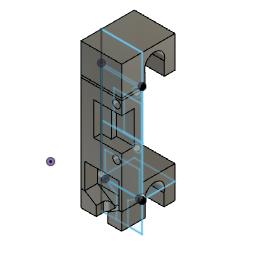
X Stop-block (Autodesk Fusion 360 design; units mm, degrees)
Autodesk Fusion 360 part; units mm, degrees
sketch "Sketch1" plane through (0, 0, 0) normal (1, 0, 0) x (0, 1, 0) in component "Component"
  line L0 (0, 0) -> (1, 0)
  line L1 (1, 0) -> (1, 40)
  line L2 (1, 40) -> (0, 40)
  line L3 (0, 40) -> (0, 0)
  dimension "d3" = 1
  dimension "d4" = 40
  constraint horizontal L0
  constraint vertical L1
  constraint horizontal L2
  constraint vertical L3
  constraint coincident L0.start L3.end
  measures "d3" distance of L0.start L0.end
  measures "d4" distance of L0.start L2.end
extrude "Extrude1" add sketch "Sketch1" against normal blind 20 makes body 1 in component "Component"
sketch "Sketch2" plane through (0, 1, 0) normal (0, 1, 0) x (-1, 0, 0) in component "Component"
  line L0 (0, 40) -> (0, 0)
  line L1 (0, 0) -> (20, 0)
  line L2 (20, 0) -> (20, 40)
  line L3 (20, 40) -> (0, 40)
  line L4 (6.0137, 29.6802) -> (6.0137, 12.583)
  line L5 (14.1333, 29.3642) -> (14.1333, 12.3406)
  arc A0 (14.1333, 29.3642) -> (6.0137, 29.6802) centre (10.1692, 31.9811) ccw
  line L6 (5.8481, 7.6926) -> (5.8481, 0)
  line L7 (13.9529, 7.3662) -> (13.9529, 0)
  arc A1 (6.0137, 12.583) -> (5.8481, 7.6926) centre (10, 10) ccw
  arc A2 (13.9529, 7.3662) -> (14.1333, 12.3406) centre (10, 10) ccw
  point P0 (10, 10)
  dimension "d7" = 9.5
  dimension "d8" = 9.5
  constraint coincident P0 A1.centre
  constraint vertical L4
  constraint parallel L2 L5
  constraint coincident L1 L6.end
  constraint perpendicular L1 L6
  constraint coincident L7.start A1
  constraint coincident L1 L7.end
  constraint perpendicular L1 L7
  constraint concentric A1 A2
  measures "d7" diameter of A0
  measures "d8" diameter of A1
extrude "Extrude2" cut sketch "Sketch2" against normal up to surface (1 mm away) contours L1 L4 L5 A0 L6 L7 A1 A2 bodies 1 in component "Component"
extrude "Extrude3" add 1 faces at (-18.2048, 0, 17.0423) along direction (0, -1, 0) blind 4 on bodies 1 bodies 1 in component "Component"
extrude "Extrude4" add 1 faces at (-20, -2.3333, 26.6667) along direction (-1, 0, 0) blind 13 on bodies 1 bodies 1 in component "Component"
sketch "Sketch3" plane through (0, 0, 40) normal (0, 0, 1) x (-1, 0, 0)
  line L0 (0, 4) -> (0, -1)
  line L1 (0, -1) -> (33, -1)
  line L2 (33, -1) -> (33, 4)
  line L3 (33, 4) -> (0, 4)
  line L4 (33, -1) -> (17, -1)
  line L5 (17, -1) -> (17, 4)
  line L6 (17, 4) -> (33, 4)
  line L7 (33, 4) -> (33, -1)
  dimension "d16" = 16
  constraint horizontal L4
  constraint vertical L5
  constraint horizontal L6
  constraint vertical L7
  constraint coincident L1.end L2.start
  measures "d16" distance of L1.end L4.end
extrude "Extrude5" add sketch "Sketch3" along normal blind 28 contours L1 L2 L3 L4 L5 L6 L7 bodies 1 in component "Component"
sketch "Sketch4" plane through (0, -4, 0) normal (0, -1, 0) x (1, 0, 0)
  line L0 (-13.9529, 0) -> (-13.9529, 7.3662)
  arc A0 (-14.1333, 12.3406) -> (-13.9529, 7.3662) centre (-10, 10) ccw
  line L1 (-14.1333, 12.3406) -> (-14.1333, 29.3642)
  arc A1 (-6.0137, 29.6802) -> (-14.1333, 29.3642) centre (-10.1692, 31.9811) ccw
  line L2 (-6.0137, 29.6802) -> (-6.0137, 12.583)
  arc A2 (-5.8481, 7.6926) -> (-6.0137, 12.583) centre (-10, 10) ccw
  line L3 (-5.8481, 7.6926) -> (-5.8481, 0)
  line L4 (-5.8481, 0) -> (0, 0)
  line L5 (0, 0) -> (0, 40)
  line L6 (0, 40) -> (-17, 40)
  line L7 (-17, 40) -> (-17, 68)
  line L8 (-17, 68) -> (-33, 68)
  line L9 (-33, 68) -> (-33, 0)
  line L10 (-33, 0) -> (-13.9529, 0)
  line L11 (-20, 0) -> (-20, 20)
  line L12 (-20, 20) -> (-33, 29.3642)
  line L13 (-33, 0) -> (-20, 0)
  line L14 (-33, 29.3642) -> (-33, 0)
  constraint coincident L10 L11.start
  constraint perpendicular L10 L11
  constraint coincident L9 L12.end
  constraint coincident L9.end L10.start
extrude "Extrude6" cut sketch "Sketch4" against normal up to surface (5 mm away) contours L9 L10 L11 L12 L13 L14 bodies 1 in component "Component"
fillet "Fillet2" radius 32.5 1 edges at (-20, -1.5, 20) on bodies 1 in component "Component"
sketch "Sketch5" plane through (0, 1, 0) normal (0, 1, 0) x (-1, 0, 0)
  line L0 (20, 0) -> (20, 3.3642)
  arc A0 (33, 29.3642) -> (20, 3.3642) centre (52.5, 3.3642) ccw
  line L1 (33, 29.3642) -> (33, 68)
  line L2 (33, 68) -> (17, 68)
  line L3 (17, 68) -> (17, 40)
  line L4 (0, 40) -> (0, 0)
  line L5 (0, 0) -> (5.8481, 0)
  line L6 (5.8481, 0) -> (5.8481, 7.6926)
  arc A1 (6.0137, 12.583) -> (5.8481, 7.6926) centre (10, 10) ccw
  line L7 (6.0137, 12.583) -> (6.0137, 29.6802)
  arc A2 (14.1333, 29.3642) -> (6.0137, 29.6802) centre (10.1692, 31.9811) ccw
  line L8 (14.1333, 29.3642) -> (14.1333, 12.3406)
  arc A3 (13.9529, 7.3662) -> (14.1333, 12.3406) centre (10, 10) ccw
  line L9 (13.9529, 7.3662) -> (13.9529, 0)
  line L10 (13.9529, 0) -> (20, 0)
  line L11 (17, 40) -> (0, 40)
sketch "Sketch6" plane through (0, -4, 0) normal (0, -1, 0) x (1, 0, 0)
  line L0 (-20, 3.3642) -> (-20, 0)
  line L1 (-20, 0) -> (-13.9529, 0)
  line L2 (-13.9529, 0) -> (-13.9529, 7.3662)
  arc A0 (-14.1333, 12.3406) -> (-13.9529, 7.3662) centre (-10, 10) ccw
  line L3 (-14.1333, 12.3406) -> (-14.1333, 29.3642)
  arc A1 (-6.0137, 29.6802) -> (-14.1333, 29.3642) centre (-10.1692, 31.9811) ccw
  line L4 (-6.0137, 29.6802) -> (-6.0137, 12.583)
  arc A2 (-5.8481, 7.6926) -> (-6.0137, 12.583) centre (-10, 10) ccw
  line L5 (-5.8481, 7.6926) -> (-5.8481, 0)
  line L6 (-5.8481, 0) -> (0, 0)
  line L7 (0, 0) -> (0, 40)
  line L8 (-17, 40) -> (-17, 68)
  line L9 (-17, 68) -> (-33, 68)
  line L10 (-33, 68) -> (-33, 29.3642)
  arc A3 (-20, 3.3642) -> (-33, 29.3642) centre (-52.5, 3.3642) ccw
  line L11 (-17, 68) -> (-33, 68)
  line L12 (-33, 68) -> (-33, 62)
  line L13 (-17, 62) -> (-17, 68)
  line L14 (-17, 62) -> (-24, 62)
  line L15 (-24, 62) -> (-24, 49)
  line L16 (-24, 49) -> (-17, 49)
  line L17 (-17, 49) -> (-17, 62)
  line L18 (0, 40) -> (-17, 40)
  line L19 (-24, 39.2) -> (-17, 39.2)
  line L20 (-17, 39.2) -> (-31.5, 39.2)
  line L21 (-31.5, 39.2) -> (-31.5, 29.2)
  line L22 (-31.5, 29.2) -> (-17, 29.2)
  line L23 (-17, 29.2) -> (-17, 39.2)
  dimension "d25" = 6
  dimension "d26" = 7
  dimension "d27" = 13
  dimension "d28" = 9.8
  dimension "d30" = 10
  constraint horizontal L11
  constraint vertical L12
  constraint vertical L13
  constraint coincident L8.end L9.start
  constraint horizontal L14
  constraint vertical L15
  constraint horizontal L16
  constraint vertical L17
  constraint horizontal L19
  constraint horizontal L20
  constraint vertical L21
  constraint horizontal L22
  constraint vertical L23
  measures "d25" distance of L8.end L13.start
  measures "d26" distance of L13.start L14.end
  measures "d27" distance of L13.start L16.end
  measures "d28" distance of L15.end L19.start
  measures "d30" distance of L19.end L22.end
extrude "Extrude7" cut sketch "Sketch6" against normal blind 2 contours L8 L14 L15 L16 L17 | L19 L20 L21 L22 L23 bodies 1 in component "Component"
sketch "Sketch7" plane through (0, -4, 0) normal (0, -1, 0) x (1, 0, 0)
  line L0 (-24, 62) -> (-17, 62)
  line L1 (-17, 62) -> (-17, 68)
  line L2 (-17, 68) -> (-33, 68)
  line L3 (-33, 68) -> (-33, 29.3642)
  arc A0 (-20, 3.3642) -> (-33, 29.3642) centre (-52.5, 3.3642) ccw
  line L4 (-20, 3.3642) -> (-20, 0)
  line L5 (-20, 0) -> (-13.9529, 0)
  line L6 (-13.9529, 0) -> (-13.9529, 7.3662)
  arc A1 (-14.1333, 12.3406) -> (-13.9529, 7.3662) centre (-10, 10) ccw
  line L7 (-14.1333, 12.3406) -> (-14.1333, 29.3642)
  arc A2 (-6.0137, 29.6802) -> (-14.1333, 29.3642) centre (-10.1692, 31.9811) ccw
  line L8 (-6.0137, 29.6802) -> (-6.0137, 12.583)
  arc A3 (-5.8481, 7.6926) -> (-6.0137, 12.583) centre (-10, 10) ccw
  line L9 (-5.8481, 7.6926) -> (-5.8481, 0)
  line L10 (-5.8481, 0) -> (0, 0)
  line L11 (0, 0) -> (0, 40)
  line L12 (0, 40) -> (-17, 40)
  line L13 (-17, 40) -> (-17, 49)
  line L14 (-17, 49) -> (-24, 49)
  line L15 (-24, 49) -> (-24, 62)
  line L16 (-31.5, 39.2) -> (-17, 39.2)
  line L17 (-17, 39.2) -> (-17, 29.2)
  line L18 (-17, 29.2) -> (-31.5, 29.2)
  line L19 (-31.5, 29.2) -> (-31.5, 39.2)
  line L20 (-24, 62) -> (-28, 62)
  line L21 (-28, 62) -> (-28, 49)
  line L22 (-28, 49) -> (-24, 49)
  line L23 (-24, 49) -> (-24, 62)
  line L24 (-33, 39.2) -> (-33, 68)
  line L25 (-17, 68) -> (-17, 62)
  line L26 (-28, 49) -> (-17, 49)
  line L27 (-17, 39.2) -> (-31.5, 39.2)
  line L28 (-31.5, 29.2) -> (-33, 29.3642)
  line L29 (0, 29.6802) -> (-6.0137, 29.6802)
  line L30 (-14.1333, 29.3642) -> (-17, 29.3642)
  dimension "d33" = 4
  constraint horizontal L20
  constraint vertical L21
  constraint horizontal L22
  constraint vertical L23
  constraint coincident L0.start L15.end
  constraint coincident L16.start L19.end
  constraint coincident L3 L24.start
  constraint coincident L2.end L3.start
  constraint coincident L1.end L2.start
  constraint coincident L0.end L1.start
  constraint coincident L13.end L14.start
  constraint coincident L16.end L17.start
  constraint coincident L18.end L19.start
  constraint coincident L3.end A0.end
  constraint coincident L11 L29.start
  constraint coincident A2.start L8.start
  constraint perpendicular L8 L29
  constraint coincident L7.end A2.end
  constraint coincident L17 L30.end
  constraint perpendicular L17 L30
  measures "d33" distance of L0.start L20.end
extrude "Extrude8" add sketch "Sketch7" along normal blind 3 contours L0 L1 L2 L3 A2 L11 L12 L13 L14 L16 L17 L19 L20 L21 L22 L24 L25 L26 L27 L28 L29 L30 bodies 1 in component "Component"
fillet "Fillet3" radius 3 2 edges at (-3.0068, -4, 29.6802) (-15.5667, -4, 29.3642) on bodies 1 in component "Component"
extrude "Extrude9" add 6 faces at (-17, -5, 33.5326) (-17, -5, 38.0056) (-17, -4.6737, 29.2547) (-17, -2.6667, 31.3937) (-17, -3.3333, 36.8112) (-17, -4.5494, 28.6794) along direction (-1, 0, 0) blind 1 on bodies 1 bodies 1 in component "Component"
sketch "Sketch8" plane through (0, -7, 0) normal (0, -1, 0) x (1, 0, 0)
  line L0 (0, 29.6802) -> (0, 40)
  line L1 (0, 40) -> (-17, 40)
  line L2 (-17, 40) -> (-17, 49)
  line L3 (-17, 49) -> (-28, 49)
  line L4 (-28, 49) -> (-28, 62)
  line L5 (-28, 62) -> (-17, 62)
  line L6 (-17, 62) -> (-17, 68)
  line L7 (-17, 68) -> (-33, 68)
  line L8 (-33, 68) -> (-33, 39.2)
  line L9 (-33, 39.2) -> (-33, 29.3642)
  line L10 (-33, 29.3642) -> (-31.5, 29.2)
  line L11 (-31.5, 29.2) -> (-31.5, 39.2)
  line L12 (-31.5, 39.2) -> (-18, 39.2)
  line L13 (-18, 39.2) -> (-18, 29.3642)
  line L14 (-18, 29.3642) -> (-14.1333, 29.3642)
  arc A0 (-6.0137, 29.6802) -> (-14.1333, 29.3642) centre (-10.1692, 31.9811) ccw
  line L15 (-6.0137, 29.6802) -> (0, 29.6802)
  circle A1 centre (-19, 65) radius 1.5
  circle A2 centre (-19, 46) radius 1.5
  dimension "d42" = 3
  dimension "d44" = 3
  measures "d42" diameter of A1
  measures "d44" diameter of A2
extrude "Extrude10" cut sketch "Sketch8" against normal up to surface (8 mm away) contours A1 | A2 bodies 1 in component "Component"
fillet "Fillet4" radius 0.5 tangency weight 0.94957 1 edges at (-32.25, -4, 29.2821) on bodies 1 in component "Component"
sketch "Sketch9" plane through (0, -7, 0) normal (0, -1, 0) x (1, 0, 0)
  circle A0 centre (-19, 65) radius 1.5
  circle A1 centre (-19, 46) radius 1.5
  line L0 (0, 29.6802) -> (0, 40)
  line L1 (0, 40) -> (-17, 40)
  line L2 (-17, 40) -> (-17, 49)
  line L3 (-17, 49) -> (-28, 49)
  line L4 (-28, 49) -> (-28, 62)
  line L5 (-28, 62) -> (-17, 62)
  line L6 (-17, 62) -> (-17, 68)
  line L7 (-17, 68) -> (-33, 68)
  line L8 (-33, 68) -> (-33, 39.2)
  line L9 (-33, 39.2) -> (-33, 29.3642)
  line L10 (-33, 29.3642) -> (-31.5, 29.2)
  line L11 (-31.5, 29.2) -> (-31.5, 39.2)
  line L12 (-31.5, 39.2) -> (-18, 39.2)
  line L13 (-18, 39.2) -> (-18, 29.3642)
  line L14 (-18, 29.3642) -> (-14.1333, 29.3642)
  arc A2 (-6.0137, 29.6802) -> (-14.1333, 29.3642) centre (-10.1692, 31.9811) ccw
  line L15 (-6.0137, 29.6802) -> (0, 29.6802)
  line L16 (-17, 40, 0) -> (-17.6105, 7.0787, -4.8416)
  line L17 (-17.6105, 7.0787, -4.8416) -> (-18.5087, 7.0787, -4.7856)
  constraint coincident L1.end L2.start
sketch "Sketch10" plane through (0, -7, 0) normal (0, -1, 0) x (1, 0, 0)
sketch "SensorHold" plane through (0, -7, 0) normal (0, -1, 0) x (1, 0, 0) in component "Sensor mount"
  line L0 (19.9806, 43.6177, -7) -> (35.9806, 43.6177, -7)
  line L1 (35.9806, 43.6177, -7) -> (35.9806, 4.8177, -7)
  line L2 (35.9806, 4.8177, -7) -> (19.9806, 4.8177, -7)
  line L3 (19.9806, 4.8177, -7) -> (19.9806, 43.6177, -7)
  line L4 (24.9806, 37.6177, -7) -> (35.9806, 37.6177, -7)
  line L5 (35.9806, 37.6177, -7) -> (35.9806, 24.6177, -7)
  line L6 (35.9806, 24.6177, -7) -> (24.9806, 24.6177, -7)
  line L7 (24.9806, 24.6177, -7) -> (24.9806, 37.6177, -7)
  line L8 (28.9806, 37.6177, -7) -> (35.9806, 37.6177, -7)
  line L9 (35.9806, 37.6177, -7) -> (35.9806, 24.6177, -7)
  line L10 (35.9806, 24.6177, -7) -> (28.9806, 24.6177, -7)
  line L11 (28.9806, 24.6177, -7) -> (28.9806, 37.6177, -7)
  line L12 (21.4806, 14.8177, -7) -> (34.9806, 14.8177, -7)
  line L13 (34.9806, 14.8177, -7) -> (34.9806, 4.8177, -7)
  line L14 (34.9806, 4.8177, -7) -> (21.4806, 4.8177, -7)
  line L15 (21.4806, 4.8177, -7) -> (21.4806, 14.8177, -7)
  circle A0 through (35.4806, 40.6177, -7) (33.2306, 41.9168, -7) (33.2306, 39.3187, -7)
  circle A1 through (35.4806, 21.6177, -7) (33.2306, 22.9168, -7) (33.2306, 20.3187, -7)
  dimension "d55" = 10
  dimension "d56" = 38.8
extrude "Extrude1'" add sketch "SensorHold" along normal blind 3 separate body contours L1 L4 L5 L6 L8 L9 L10 L11 | L2 L12 L13 L14 L15 in plane through (0, 0, 0) normal (0, -1, 0) makes body 2 at (31.3139, 0, 33.2844) makes body 3 at (25.9806, 0, 11.4844) in component "Sensor mount"
extrude "Extrude2'" add sketch "SensorHold" along normal blind 5 contours L4 L6 L7 L11 in plane through (0, 0, 0) normal (0, -1, 0) bodies 2 in component "Sensor mount"
extrude "Extrude3'" add sketch "SensorHold" along normal blind 8 contours L0 L1 L2 L3 L4 L6 L7 L8 L10 L12 L13 L15 in plane through (0, 0, 0) normal (0, -1, 0) bodies 2 3 in component "Sensor mount"
sketch "Sketch1 (2)" plane through (0, 0, 0) normal (0, 1, 0) x (1, 0, 0) in component "On Print Mount"
  line L0 (35.9806, -42.7177) -> (35.9806, -24.2177)
  line L1 (19.9806, -4.8177) -> (19.9806, -43.6177)
  line L2 (35.9806, -24.2177) -> (36, -24.2177)
  line L3 (36, -24.2177) -> (36, -55.2177)
  line L4 (36, -55.2177) -> (19.9806, -55.2177)
  line L5 (19.9806, -55.2177) -> (19.9806, -24.2177)
  line L6 (35.9806, -24.2177) -> (36, -24.2177)
  line L7 (36, -24.2177) -> (36, 6.7823)
  line L8 (36, 6.7823) -> (19.9806, 6.7823)
  line L9 (19.9806, 6.7823) -> (19.9806, -24.2177)
  line L10 (19.9806, -24.2177) -> (36, -24.2177)
  line L11 (36, -24.2177) -> (36, -42.7177)
  line L12 (36, -42.7177) -> (19.9806, -42.7177)
  line L13 (19.9806, -42.7177) -> (19.9806, -24.2177)
  line L14 (19.9806, -24.2177) -> (36, -24.2177)
  line L15 (36, -24.2177) -> (36, -5.7177)
  line L16 (36, -5.7177) -> (35.9806, -5.7177)
  line L17 (19.9806, -5.7177) -> (19.9806, -24.2177)
  line L18 (21.4806, -4.8177) -> (25.9801, -1.9974)
  line L19 (34.9806, -4.8177) -> (30.481, -1.9974)
  line L20 (30.481, -1.9974) -> (30.481, 6.7823)
  line L21 (25.9801, -1.9974) -> (25.9801, 6.7823)
  line L22 (21.4806, -4.8177) -> (34.9806, -4.8177)
  line L23 (21.4806, -4.8177) -> (19.9806, -4.8177)
  line L24 (34.9806, -4.8177) -> (35.9806, -4.8177)
  line L25 (35.9806, -4.8177) -> (36, -4.8177)
  line L26 (35.9806, -43.6177) -> (36, -43.6177)
  line L27 (36, -55.2177) -> (19.9806, -55.2177)
  point P0 (19.9806, -43.6177)
  point P1 (35.9806, -43.6177)
  point P2 (35.9806, -4.8177)
  point P3 (21.4806, -4.8177)
  point P4 (34.9806, -4.8177)
  dimension "d59" = 31
  dimension "d60" = 31
  dimension "d61" = 18.5
  dimension "d62" = 18.5
  constraint vertical L0
  constraint vertical L1
  constraint coincident P0 L1.end
  constraint coincident L24.end L25.start
  constraint horizontal L2
  constraint vertical L3
  constraint horizontal L4
  constraint vertical L5
  constraint midpoint L1 L5.end
  constraint horizontal L6
  constraint vertical L7
  constraint horizontal L8
  constraint vertical L9
  constraint horizontal L10
  constraint vertical L11
  constraint horizontal L12
  constraint vertical L13
  constraint horizontal L14
  constraint vertical L15
  constraint horizontal L16
  constraint vertical L17
  constraint coincident P3 L18.start
  constraint coincident P4 L19.start
  constraint coincident L8 L20.end
  constraint perpendicular L8 L20
  constraint coincident L8 L21.end
  constraint perpendicular L8 L21
  constraint coincident P2 L24.end
  constraint coincident L7 L25.end
  constraint perpendicular L7 L25
  constraint coincident L12 L0.start
  constraint coincident P1 L26.start
  constraint coincident L3 L26.end
  constraint perpendicular L3 L26
  measures "d59" distance of L5.end L4.end
  measures "d60" distance of L5.end L8.end
  measures "d61" distance of L5.end L12.end
  measures "d62" distance of L5.end L17.start
extrude "Extrude1''" add sketch "Sketch1 (2)" against normal up to surface (8 mm away) separate body contours L1 L3 L4 L5 L12 L27 | L7 L8 L19 L20 L24 L25 | L8 L9 L18 L21 L23 makes body 4 at (19.9806, -2.6667, -2.9156) makes body 5 at (36, -2.6667, 0.9511) makes body 6 at (25.3204, 0, 46.8844) in component "On Print Mount"
extrude "Extrude2''" add sketch "Sketch1 (2)" against normal up to surface (3 mm away) contours L8 L18 L19 L20 L21 L22 bodies 4 5 in component "On Print Mount"
extrude "Extrude3''" add sketch "Sketch1 (2)" along normal blind 13 contours L1 L3 L4 L5 L12 L27 | L7 L8 L19 L20 L24 L25 | L8 L9 L18 L21 L23 | L8 L18 L19 L20 L21 L22 bodies 4 6 in component "On Print Mount"
sketch "Sketch5 (2)" plane through (19.9806, 0, 0) normal (-1, 0, 0) x (0, -1, 0) in component "On Print Mount"
  line L0 (8, 42.7177) -> (8, 55.2177)
  line L1 (8, 55.2177) -> (-13, 55.2177)
  line L2 (-13, 55.2177) -> (-13, 42.7177)
  line L3 (-13, 42.7177) -> (8, 42.7177)
sketch "Sketch6 (2)" plane through (0, 0, 4.8177) normal (0, 0, 1) x (-1, 0, 0) in component "On Print Mount"
  line L0 (-21.4806, 3) -> (-34.9806, 3)
  line L1 (-34.9806, 3) -> (-34.9806, -13)
  line L2 (-34.9806, -13) -> (-21.4806, -13)
  line L3 (-21.4806, -13) -> (-21.4806, 3)
  line L4 (-20, 0) -> (-36, 0)
  line L5 (-20, 0) -> (-36, 0)
  line L6 (-20, -13) -> (-36, -13)
  line L7 (-36, -13) -> (-36, 0)
  line L8 (-36, 0) -> (-20, 0)
  line L9 (-20, 0) -> (-20, -13)
  constraint perpendicular L1 L4
  constraint horizontal L6
  constraint vertical L7
  constraint horizontal L8
  constraint vertical L9
extrude "Extrude4'" add sketch "Sketch6 (2)" along normal blind 6 contours L3 L4 L5 L6 L8 L9 | L1 L2 L3 L4 L5 L6 L8 | L1 L4 L5 L6 L7 L8 bodies 4 in component "On Print Mount"
sketch "Sketch7 (2)" plane through (19.9806, 2.5, 48.9677) normal (-1, 0, 0) x (0, -1, 0) in component "On Print Mount"
  line L0 (-6.3178, -1.0135) -> (-6.3178, -7.6901)
  line L1 (1.3178, -1.0135) -> (1.3178, -7.6565)
  arc A0 (1.3178, -1.0135) -> (-6.3178, -1.0135) centre (-2.5, 0) ccw
  line L2 (-6.1754, -45.947) -> (-6.1754, -56)
  line L3 (-6.1754, -56) -> (1.1754, -56)
  line L4 (1.1754, -56) -> (1.1754, -45.947)
  arc A1 (1.1754, -45.947) -> (-6.1754, -45.947) centre (-2.5, -44.5) ccw
  line L5 (-6.3178, -7.6901) -> (1.3178, -7.6565)
  dimension "d76" = 7.9
  dimension "d78" = 44.5
  dimension "d79" = 7.9
  constraint perpendicular L2 L3
  constraint vertical L0
  constraint vertical L1
  measures "d76" diameter of A0
  measures "d78" distance of A0.centre A1.centre
  measures "d79" diameter of A1
extrude "Extrude5'" cut 1 faces at (27.3202, 7.6667, -6.7823) along direction (0, 0, 1) blind 5 on bodies 4 bodies 4 in component "On Print Mount"
extrude "Extrude6'" cut sketch "Sketch7 (2)" against normal up to surface (16.0194 mm away) bodies 4 6 in component "On Print Mount"
fillet "Fillet1" radius 2.25 2 edges at (30.481, -3, 0.1076) (25.9801, -3, 0.1076) on bodies 4 in component "On Print Mount"
sketch "Sketch11" plane through (0, 0, 0) normal (0, 1, 0) x (-1, 0, 0)
move_body "Move1" [suppressed] in component "Sensor mount"
component "Component" placed x (1, 0, 0) y (0, 1, 0) z (0, 0, 1) at (0, 0, 0)
component "Sensor mount" placed x (1, 0, 0) y (0, 1, 0) z (0, 0, 1) at (0, 0, 0)
component "On Print Mount" placed x (1, 0, 0) y (0, 1, 0) z (0, 0, 1) at (0, 0, 0)
equation "d56 = 3.90 cm - 0.02 cm"
equation "d59 = ( 6.2 / 2 ) * 1 cm"
equation "d60 = ( 6.2 / 2 ) * 1 cm"
equation "d61 = ( 3.7 / 2 ) * 1 cm"
equation "d62 = ( 3.7 / 2 ) * 1 cm"
equation "d72 = 2.1 cm - 0.8 cm"
equation "d78 = 0.4 cm + 3.65 cm + 0.4 cm"
